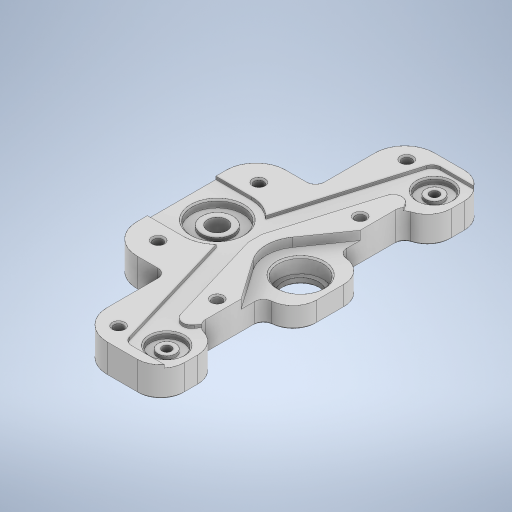
# Autodesk Inventor part: top
Saved by Autodesk Inventor 2023.1 (Build 271208000, 208)
## iProperties
Created: 2023-11-16
Part Number: top
Material: Všeobecné
Document SubType Name: Modeling
Designer: zavrel
Density: 1 g/cm^3
Appearance: Výchozí
Author: zavrel
Autodesk Inventor part; units mm, degrees
ref_plane "YZ Plane" through (0, 0, 0) normal (1, 0, 0) x (0, 1, 0)
ref_plane "XZ Plane" through (0, 0, 0) normal (0, 1, 0) x (-1, 0, 0)
ref_plane "XY Plane" through (0, 0, 0) normal (0, 0, 1) x (1, 0, 0)
sketch "Náčrt1" plane through (0, 0, 0) normal (0, 1, 0) x (-1, 0, 0)
  line L0 (-26.1298, 2.5) -> (-26.1298, 15)
  line L1 (-26.1298, 15) -> (-16.1298, 15)
  line L2 (-16.1298, 15) -> (-16.1298, 37.5)
  line L3 (-16.1298, 37.5) -> (-24.1298, 37.5)
  line L4 (-24.1298, 37.5) -> (-24.1298, 57.5)
  line L5 (-24.1298, 57.5) -> (-16.1298, 57.5)
  line L6 (-16.1298, 57.5) -> (3.8702, 57.5)
  line L7 (3.8702, 57.5) -> (3.8702, 27.5)
  line L8 (3.8702, 27.5) -> (23.8702, 27.5)
  line L9 (23.8702, 27.5) -> (23.8702, 2.5)
  line L10 (23.8702, 2.5) -> (-26.1298, 2.5) construction
  line L11 (-26.1298, 2.5) -> (-26.1298, -10)
  line L12 (-26.1298, -10) -> (-16.1298, -10)
  line L13 (-16.1298, -10) -> (-16.1298, -32.5)
  line L14 (-16.1298, -32.5) -> (-24.1298, -32.5)
  line L15 (-24.1298, -32.5) -> (-24.1298, -52.5)
  line L16 (-24.1298, -52.5) -> (-16.1298, -52.5)
  line L17 (-16.1298, -52.5) -> (3.8702, -52.5)
  line L18 (3.8702, -52.5) -> (3.8702, -22.5)
  line L19 (3.8702, -22.5) -> (23.8702, -22.5)
  line L20 (23.8702, -22.5) -> (23.8702, 2.5)
  circle A0 centre (-16.1298, 47.5) radius 5.5
  line L21 (-24.1298, 47.5) -> (17.4251, 47.5) construction
  circle A1 centre (-16.1298, -42.5) radius 5.5
  line L22 (-24.1298, -42.5) -> (17.4251, -42.5) construction
  circle A2 centre (11.8702, 2.5) radius 8.5
  circle A3 centre (-16.1298, 2.5) radius 7.5
  line L23 (-16.1298, 47.5) -> (-16.1298, -42.5) construction
  point P0 (0, 0)
  point P1 (-26.1298, 8.75)
  point P2 (-16.1298, 2.5)
  dimension "d0" = 25
  dimension "d1" = 50
  dimension "d3" = 20
  dimension "d4" = 8
  dimension "d5" = 20
  dimension "d6" = 20
  dimension "d7" = 11
  dimension "d8" = 90
  dimension "d9" = 8
  dimension "d10" = 17
  dimension "d13" = 15
  dimension "d15" = 12
  dimension "d17" = 10
  constraints: 48 end point, 12 symmetric about line, 9 perpendicular, 8 point on line, 4 centre point, 4 midpoint, 2 vertical, 1 horizontal, 1 other
  measures "d0" distance between parallel lines of L12 L1
  measures "d1" distance between parallel lines of L19 L8
  measures "d3" distance of L3.end L4.end
  measures "d4" distance between parallel lines of L13 L15
  measures "d5" distance between parallel lines of L13 L18
  measures "d6" distance between parallel lines of L18 L20
  measures "d7" diameter of A0
  measures "d8" distance of L23.end L23.start
  measures "d9" distance from line of L4 L23.start
  measures "d10" diameter of A2
  measures "d13" diameter of A3
  measures "d15" distance from line of L9 A2.centre
  measures "d17" distance of L11.end L12.end
extrude "Vysunutí1" add sketch "Náčrt1" along normal blind 10
sketch "Náčrt2" plane through (0, 0, 0) normal (0, -1, 0) x (1, 0, 0)
  line L0 (16.1298, -10) -> (16.1298, -32.5) projected
  line L1 (26.1298, -10) -> (16.1298, -10) projected
  line L2 (26.1298, 15) -> (26.1298, -10) projected
  line L3 (16.1298, 15) -> (26.1298, 15) projected
  line L4 (16.1298, 37.5) -> (16.1298, 15) projected
  line L5 (24.1298, 37.5) -> (16.1298, 37.5) projected
  line L6 (24.1298, 57.5) -> (24.1298, 37.5) projected
  line L7 (-3.8702, 57.5) -> (24.1298, 57.5) projected
  line L8 (-3.8702, 27.5) -> (-3.8702, 57.5) projected
  line L9 (-23.8702, 27.5) -> (-3.8702, 27.5) projected
  line L10 (-23.8702, -22.5) -> (-23.8702, 27.5) projected
  line L11 (-3.8702, -22.5) -> (-23.8702, -22.5) projected
  line L12 (-3.8702, -52.5) -> (-3.8702, -22.5) projected
  line L13 (24.1298, -52.5) -> (-3.8702, -52.5) projected
  line L14 (24.1298, -32.5) -> (24.1298, -52.5) projected
  line L15 (16.1298, -32.5) -> (24.1298, -32.5) projected
  circle A0 centre (16.1298, 47.5) radius 5.5 projected
  circle A1 centre (16.1298, -42.5) radius 5.5 projected
  circle A2 centre (-11.8702, 2.5) radius 8.5 projected
  circle A3 centre (16.1298, 2.5) radius 7.5 projected
  circle A4 centre (16.1298, -42.5) radius 1.5
  circle A5 centre (16.1298, 47.5) radius 5.5 projected
  circle A6 centre (16.1298, 47.5) radius 1.5
  point P0 (0, 0)
  dimension "d20" = 3
  constraints: 2 centre point, 2 coincident, 1 equal radius
  measures "d20" diameter of A6
extrude "Vysunutí2" add sketch "Náčrt2" against normal blind 8 contours A0 | A1
sketch "Náčrt3" plane through (0, 0, 0) normal (0, -1, 0) x (1, 0, 0)
  circle A0 centre (16.1298, 47.5) radius 1.5 projected
  circle A1 centre (16.1298, -42.5) radius 1.5 projected
  line L0 (16.1298, -10) -> (16.1298, -32.5) projected
  line L1 (26.1298, -10) -> (16.1298, -10) projected
  line L2 (26.1298, 15) -> (26.1298, -10) projected
  line L3 (16.1298, 15) -> (26.1298, 15) projected
  line L4 (16.1298, 37.5) -> (16.1298, 15) projected
  line L5 (24.1298, 37.5) -> (16.1298, 37.5) projected
  line L6 (24.1298, 57.5) -> (24.1298, 37.5) projected
  line L7 (-3.8702, 57.5) -> (24.1298, 57.5) projected
  line L8 (-3.8702, 27.5) -> (-3.8702, 57.5) projected
  line L9 (-23.8702, 27.5) -> (-3.8702, 27.5) projected
  line L10 (-23.8702, -22.5) -> (-23.8702, 27.5) projected
  line L11 (-3.8702, -22.5) -> (-23.8702, -22.5) projected
  line L12 (-3.8702, -52.5) -> (-3.8702, -22.5) projected
  line L13 (24.1298, -52.5) -> (-3.8702, -52.5) projected
  line L14 (24.1298, -32.5) -> (24.1298, -52.5) projected
  line L15 (16.1298, -32.5) -> (24.1298, -32.5) projected
  circle A2 centre (-11.8702, 2.5) radius 8.5 projected
  circle A3 centre (16.1298, 2.5) radius 7.5 projected
  circle A4 centre (16.1298, 2.5) radius 6
  point P0 (0, 0)
  dimension "d24" = 12
  constraints: 1 centre point, 1 coincident
  measures "d24" diameter of A4
extrude "Vysunutí3" add sketch "Náčrt3" against normal blind 2 contours A3
sketch "Náčrt4" plane through (0, 0, 0) normal (0, -1, 0) x (1, 0, 0)
  circle A0 centre (16.1298, 2.5) radius 6 projected
  circle A1 centre (16.1298, 47.5) radius 1.5 projected
  circle A2 centre (16.1298, -42.5) radius 1.5 projected
  line L0 (16.1298, -10) -> (16.1298, -32.5) projected
  line L1 (26.1298, -10) -> (16.1298, -10) projected
  line L2 (26.1298, 15) -> (26.1298, -10) projected
  line L3 (16.1298, 15) -> (26.1298, 15) projected
  line L4 (16.1298, 37.5) -> (16.1298, 15) projected
  line L5 (24.1298, 37.5) -> (16.1298, 37.5) projected
  line L6 (24.1298, 57.5) -> (24.1298, 37.5) projected
  line L7 (-3.8702, 57.5) -> (24.1298, 57.5) projected
  line L8 (-3.8702, 27.5) -> (-3.8702, 57.5) projected
  line L9 (-23.8702, 27.5) -> (-3.8702, 27.5) projected
  line L10 (-23.8702, -22.5) -> (-23.8702, 27.5) projected
  line L11 (-3.8702, -22.5) -> (-23.8702, -22.5) projected
  line L12 (-3.8702, -52.5) -> (-3.8702, -22.5) projected
  line L13 (24.1298, -52.5) -> (-3.8702, -52.5) projected
  line L14 (24.1298, -32.5) -> (24.1298, -52.5) projected
  line L15 (16.1298, -32.5) -> (24.1298, -32.5) projected
  circle A3 centre (-11.8702, 2.5) radius 8.5 projected
  circle A4 centre (-11.8702, 2.5) radius 3.25
  point P0 (0, 0)
  dimension "d27" = 6.5
  constraints: 1 centre point, 1 coincident
  measures "d27" diameter of A4
extrude "Vysunutí4" add sketch "Náčrt4" against normal blind 7.5 contours A3
sketch "Náčrt5" plane through (-11.8702, 7.5, 2.5) normal (0, 1, 0) x (1, 0, 0)
  circle A0 centre (0, 0) radius 8.5 projected
  circle A1 centre (0, 0) radius 3.25 projected
  circle A2 centre (0, 0) radius 3.25 projected
  circle A3 centre (0, 0) radius 5.25
  point P0 (11.8702, 2.5)
  dimension "d68" = 2
  constraints: 1 centre point, 1 coincident
  measures "d68" radial gap between concentric circles of A3 A1
extrude "Vysunutí5" cut sketch "Náčrt5" against normal blind 1 contours A0
sketch "Náčrt6" plane through (16.1298, 8, -42.5) normal (0, 1, 0) x (1, 0, 0)
  circle A0 centre (0, -90) radius 5.5 projected
  circle A1 centre (0, -90) radius 1.5 projected
  circle A2 centre (0, 0) radius 5.5 projected
  circle A3 centre (0, 0) radius 1.5 projected
  circle A4 centre (0, -90) radius 1.5 projected
  circle A5 centre (0, -90) radius 3
  circle A6 centre (0, 0) radius 1.5 projected
  circle A7 centre (0, 0) radius 3
  point P0 (-16.1298, -42.5)
  dimension "d33" = 1.5
  constraints: 2 centre point, 2 coincident, 1 equal radius
  measures "d33" radial gap between concentric circles of A5 A1
extrude "Vysunutí6" cut sketch "Náčrt6" against normal blind 1 contours A0 | A2
sketch "Náčrt7" plane through (0, 10, 0) normal (0, 1, 0) x (1, 0, 0)
  line L0 (16.1298, 10) -> (16.1298, 32.5) projected
  line L1 (16.1298, 32.5) -> (24.1298, 32.5) projected
  line L2 (24.1298, 32.5) -> (24.1298, 52.5) projected
  line L3 (24.1298, 52.5) -> (-3.8702, 52.5) projected
  line L4 (-3.8702, 52.5) -> (-3.8702, 22.5) projected
  line L5 (-3.8702, 22.5) -> (-23.8702, 22.5) projected
  line L6 (-23.8702, 22.5) -> (-23.8702, -27.5) projected
  line L7 (-23.8702, -27.5) -> (-3.8702, -27.5) projected
  line L8 (-3.8702, -27.5) -> (-3.8702, -57.5) projected
  line L9 (-3.8702, -57.5) -> (24.1298, -57.5) projected
  line L10 (24.1298, -57.5) -> (24.1298, -37.5) projected
  line L11 (24.1298, -37.5) -> (16.1298, -37.5) projected
  line L12 (16.1298, -37.5) -> (16.1298, -15) projected
  line L13 (16.1298, -15) -> (26.1298, -15) projected
  line L14 (26.1298, -15) -> (26.1298, 10) projected
  line L15 (26.1298, 10) -> (16.1298, 10) projected
  circle A0 centre (16.1298, -47.5) radius 5.5 projected
  circle A1 centre (16.1298, 42.5) radius 5.5 projected
  circle A2 centre (-11.8702, -2.5) radius 8.5 projected
  circle A3 centre (16.1298, -2.5) radius 7.5 projected
  circle A4 centre (16.1298, -47.5) radius 5.5 construction
  line L16 (10.8583, -49.0689) -> (-3.7234, -0.0753) construction
  circle A5 centre (-11.8702, -2.5) radius 8.5 construction
  line L17 (-3.7234, -4.9247) -> (10.8583, 44.0689) construction
  circle A6 centre (16.1298, 42.5) radius 5.5 projected
  line L18 (12.2835, -43.3406) -> (0.8159, -4.8101)
  line L19 (16.1298, -37.5) -> (16.1298, -15) projected
  line L20 (16.1298, -37.5) -> (12.2835, -43.3406)
  line L21 (24.1298, 32.5) -> (24.1298, 52.5) projected
  line L22 (24.1298, -54.5) -> (9.0632, -54.5)
  circle A7 centre (-11.8702, -2.5) radius 11.5
  line L23 (9.0632, -54.5) -> (-3.9358, -10.8244)
  line L24 (0.8159, -2.5) -> (0.8159, -4.8101)
  circle A8 centre (-11.8702, -2.5) radius 3.25 construction
  line L25 (-11.8702, -2.5) -> (16.1298, -2.5) construction
  line L26 (12.2835, 38.3406) -> (0.8159, -0.1899)
  line L27 (16.1298, 32.5) -> (12.2835, 38.3406)
  line L28 (24.1298, 49.5) -> (9.0632, 49.5)
  line L29 (9.0632, 49.5) -> (-3.9358, 5.8244)
  line L30 (0.8159, -2.5) -> (0.8159, -0.1899)
  line L31 (-11.8702, -14) -> (-23.8702, -14)
  line L32 (-23.8702, 22.5) -> (-23.8702, -27.5) projected
  line L33 (-11.8702, 9) -> (-23.8702, 9)
  point P0 (0, 0)
  point P1 (-3.9358, 5.8244)
  dimension "d39" = 3
  dimension "d43" = 3
  dimension "d44" = 3
  constraints: 30 end point, 5 point on circle, 5 symmetric about line, 4 point on line, 4 tangent, 3 horizontal, 3 parallel, 1 centre point, 1 vertical, 6 other
  measures "d39" distance between parallel lines of L16 L18
  measures "d43" distance between parallel lines of L9 L22
  measures "d44" radial gap between concentric circles of A5 A7
extrude "Extrusion7" cut sketch "Náčrt7" against normal blind 1 contours L27 L26 L30 L24 L18 L20 L11 L10 L22 L23 A7 L29 L28 L2 L1 | A7 | A7 L31 L6 L33
sketch "Sketch8" plane through (0, 10, 0) normal (0, 1, 0) x (1, 0, 0)
  line L0 (16.1298, 32.5) -> (12.2835, 38.3406) projected
  line L1 (12.2835, 38.3406) -> (0.8159, -0.1899) projected
  line L2 (0.8159, -0.1899) -> (0.8159, -4.8101) projected
  line L3 (0.8159, -4.8101) -> (12.2835, -43.3406) projected
  line L4 (12.2835, -43.3406) -> (16.1298, -37.5) projected
  line L5 (16.1298, -37.5) -> (16.1298, -15) projected
  line L6 (16.1298, -15) -> (26.1298, -15) projected
  line L7 (26.1298, -15) -> (26.1298, 10) projected
  line L8 (26.1298, 10) -> (16.1298, 10) projected
  line L9 (16.1298, 10) -> (16.1298, 32.5) projected
  circle A0 centre (16.1298, -2.5) radius 7.5 projected
  circle A1 centre (16.1298, -2.5) radius 11.4868
  line L10 (16.1298, 10) -> (16.1298, 32.5) projected
  line L11 (16.1298, 17.5) -> (6.7265, 4.0973)
  line L12 (16.1298, -22.5) -> (6.7265, -9.0973)
  point P0 (0, 0)
  point P1 (18.102, 10)
  point P2 (18.102, -15)
  point P3 (26.1298, 3.152)
  point P4 (26.1298, -8.152)
  dimension "d49" = 20
  constraints: 4 end point, 2 point on circle, 2 point on line, 2 tangent, 1 centre point, 1 equal length
  measures "d49" distance of A0.centre L11.start
extrude "Extrusion8" cut sketch "Sketch8" against normal blind 3 contours L9 L8 L7 A1 L11 | A1 L7 | A1 L7 L6 L5 L12 | A0 picked at (25.2965, -2.5)
sketch "Sketch9" plane through (0, 10, 0) normal (0, 1, 0) x (1, 0, 0)
  line L0 (9.0632, 49.5) -> (24.1298, 49.5) projected
  line L1 (24.1298, 49.5) -> (24.1298, 52.5) projected
  line L2 (24.1298, 52.5) -> (-3.8702, 52.5) projected
  line L3 (-3.8702, 52.5) -> (-3.8702, 22.5) projected
  line L4 (-3.8702, 22.5) -> (-23.8702, 22.5) projected
  line L5 (-23.8702, 22.5) -> (-23.8702, 9) projected
  line L6 (-23.8702, -27.5) -> (-3.8702, -27.5) projected
  line L7 (-3.8702, -27.5) -> (-3.8702, -57.5) projected
  line L8 (-3.8702, -57.5) -> (24.1298, -57.5) projected
  line L9 (24.1298, -57.5) -> (24.1298, -54.5) projected
  line L10 (24.1298, -54.5) -> (9.0632, -54.5) projected
  line L11 (9.0632, -54.5) -> (-3.9358, -10.8244) projected
  arc A0 (-3.9358, 5.8244) -> (-11.8702, 9) centre (-11.8702, -2.5) ccw projected
  line L12 (-3.9358, 5.8244) -> (9.0632, 49.5) projected
  line L13 (16.1298, -22.5) -> (6.7265, -9.0973) projected
  arc A1 (6.7265, 4.0973) -> (6.7265, -9.0973) centre (16.1298, -2.5) ccw projected
  line L14 (6.7265, 4.0973) -> (16.1298, 17.5) projected
  line L15 (16.1298, 17.5) -> (16.1298, 32.5) projected
  line L16 (16.1298, 32.5) -> (12.2835, 38.3406) projected
  line L17 (12.2835, 38.3406) -> (0.8159, -0.1899) projected
  line L18 (0.8159, -0.1899) -> (0.8159, -4.8101) projected
  line L19 (0.8159, -4.8101) -> (12.2835, -43.3406) projected
  line L20 (12.2835, -43.3406) -> (16.1298, -37.5) projected
  line L21 (16.1298, -37.5) -> (16.1298, -22.5) projected
  circle A2 centre (16.1298, -2.5) radius 7.5 projected
  line L22 (26.1298, 10) -> (26.1298, -15) projected
  line L23 (16.1298, 10) -> (26.1298, 10) projected
  line L24 (16.1298, 17.5) -> (16.1298, 10) projected
  line L25 (6.7265, 4.0973) -> (16.1298, 17.5) projected
  arc A3 (6.7265, 4.0973) -> (6.7265, -9.0973) centre (16.1298, -2.5) ccw projected
  line L26 (16.1298, -22.5) -> (6.7265, -9.0973) projected
  line L27 (16.1298, -15) -> (16.1298, -22.5) projected
  line L28 (26.1298, -15) -> (16.1298, -15) projected
  line L29 (12.2835, -43.3406) -> (16.1298, -37.5) projected
  line L30 (0.8159, -4.8101) -> (12.2835, -43.3406) projected
  line L31 (0.8159, -0.1899) -> (0.8159, -4.8101) projected
  line L32 (12.2835, 38.3406) -> (0.8159, -0.1899) projected
  line L33 (16.1298, 32.5) -> (12.2835, 38.3406) projected
  line L34 (24.1298, 32.5) -> (16.1298, 32.5) projected
  line L35 (24.1298, 49.5) -> (24.1298, 32.5) projected
  line L36 (9.0632, 49.5) -> (24.1298, 49.5) projected
  line L37 (-3.9358, 5.8244) -> (9.0632, 49.5) projected
  arc A4 (-11.8702, -14) -> (-3.9358, -10.8244) centre (-11.8702, -2.5) ccw projected
  line L38 (9.0632, -54.5) -> (-3.9358, -10.8244) projected
  line L39 (24.1298, -54.5) -> (9.0632, -54.5) projected
  line L40 (24.1298, -37.5) -> (24.1298, -54.5) projected
  line L41 (16.1298, -37.5) -> (24.1298, -37.5) projected
  circle A5 centre (-11.8702, -2.5) radius 8.5 projected
  circle A6 centre (16.1298, 42.5) radius 5.5 projected
  circle A7 centre (16.1298, -47.5) radius 5.5 projected
  circle A8 centre (3.3734, -50.9251) radius 1.6
  circle A9 centre (12.1298, -26.5254) radius 1.6
  circle A10 centre (-14.8339, -19.4088) radius 1.6
  line L42 (-11.8702, -2.5) -> (16.1298, -2.5) construction
  circle A11 centre (3.3734, 45.9251) radius 1.6
  circle A12 centre (12.1298, 21.5254) radius 1.6
  circle A13 centre (-14.8339, 14.4088) radius 1.6
  arc A14 (-3.9358, 5.8244) -> (-11.8702, 9) centre (-11.8702, -2.5) ccw projected
  line L43 (-23.8702, 9) -> (-11.8702, 9) projected
  line L44 (-23.8702, -14) -> (-23.8702, 9) projected
  line L45 (-11.8702, -14) -> (-23.8702, -14) projected
  line L46 (-23.8702, 9) -> (-11.8702, 9) projected
  line L47 (-11.8702, -14) -> (-23.8702, -14) projected
  line L48 (-23.8702, -14) -> (-23.8702, -27.5) projected
  arc A15 (-11.8702, -14) -> (-3.9358, -10.8244) centre (-11.8702, -2.5) ccw projected
  point P0 (0, 0)
  dimension "d51" = 6.5749
  dimension "d52" = 7.2436
  dimension "d53" = 9.0363
  dimension "d54" = 8.0912
  dimension "d55" = 11.5254
  dimension "d56" = 4
  dimension "d57" = 3.2
  constraints: 6 centre point, 3 symmetric about line, 2 end point, 2 equal radius, 1 horizontal, 3 other
  measures "d51" distance from line of L8 A8.centre
  measures "d52" distance from line of L7 A8.centre
  measures "d53" distance from line of L5 A10.centre
  measures "d54" distance from line of L6 A10.centre
  measures "d55" distance from line of L28 A9.centre
  measures "d56" distance from line of A9.centre L21
  measures "d57" diameter of A10
extrude "Extrusion9" cut sketch "Sketch9" against normal up to surface (10 mm away) contours A8 | A9 | A10 | A11 | A12 | A13
fillet "Fillet1" radius 10 4 edges at (-23.8702, 5, 27.5) (-23.8702, 5, -22.5) (-3.8702, 5, 57.5) (-3.8702, 5, -52.5)
fillet "Fillet2" radius 3 6 edges at (16.1298, 3.5, -10) (16.1298, 4.5, -32.5) (16.1298, 3.5, 15) (16.1298, 4.5, 37.5) (-3.8702, 5, -22.5) (-3.8702, 5, 27.5)
fillet "Fillet3" radius 8 4 edges at (24.1298, 5, 57.5) (24.1298, 4.5, 37.5) (24.1298, 4.5, -32.5) (24.1298, 5, -52.5)
fillet "Fillet4" radius 8 2 edges at (26.1298, 3.5, 15) (26.1298, 3.5, -10)
fillet "Fillet5" radius 3 4 edges at (9.0632, 9.5, 54.5) (12.2835, 9.5, 43.3406) (12.2835, 9.5, -38.3406) (9.0632, 9.5, -49.5)
chamfer "Chamfer1" distance 0.5 angle 45 10 edges at (21.6298, 9, 47.5) (23.6298, 7, 2.5) (-3.3702, 9, 2.5) (21.6298, 9, -42.5) (1.7734, 10, 50.9251) (-16.4339, 10, 19.4088) (-16.4339, 10, -14.4088) (1.7734, 10, -45.9251) (10.5298, 10, -21.5254) (10.5298, 10, 26.5254)
sketch "Sketch10" plane through (0, 0, 0) normal (0, -1, 0) x (1, 0, 0)
  point P0 (0, 0)
sketch "Sketch11" plane through (-23.8702, 9, 14) normal (-1, 0, 0) x (0, 0, 1)
  line L0 (-26.5, -9) -> (-26.5, 1) projected
  line L1 (-26.5, -9) -> (3.5, -9) projected
  line L2 (3.5, 1) -> (3.5, -9) projected
  line L3 (0, 1) -> (3.5, 1) projected
  line L4 (0, 1) -> (0, 0) projected
  line L5 (0, 0) -> (-23, 0) projected
  line L6 (-23, 0) -> (-23, 1) projected
  line L7 (-26.5, 1) -> (-23, 1) projected
  line L8 (3.5, 1) -> (3.5, -9) construction
  line L9 (3.5, -4) -> (-26.5, -4) construction
  line L10 (-26.5, -9) -> (-26.5, 1) construction
  line L11 (-6.9545, -9) -> (-16.0455, -9) construction
  line L12 (-11.5, -9) -> (-11.5, 1) construction
  line L13 (-18.0973, 1) -> (-4.9027, 1) construction
  circle A0 centre (-0.5, -4) radius 1.6
  circle A1 centre (-22.5, -4) radius 1.6
  line L14 (-0.5, -4) -> (-0.5, -1.1985) construction
  line L15 (-0.5, -1.7373) -> (0.6314, -2.8686)
  line L16 (-0.5, -1.7373) -> (-1.6314, -2.8686)
  line L17 (-22.5, -1.7373) -> (-23.6314, -2.8686)
  line L18 (-22.5, -1.7373) -> (-21.3686, -2.8686)
  point P0 (-14, -9)
  point P1 (-21.3686, -2.8686)
  dimension "d69" = 3.2
  dimension "d70" = 22
  dimension "d91" = 90
  constraints: 14 end point, 4 midpoint, 4 symmetric about line, 2 centre point, 2 point on circle, 2 point on line, 2 tangent, 1 vertical, 1 other
  measures "d69" diameter of A0
  measures "d70" distance of A1.centre L14.start
  measures "d91" angle of L16 L15
sketch "Sketch12" plane through (0, 0, 0) normal (0, -1, 0) x (1, 0, 0)
  arc A0 (18.8571, -10.0124) -> (26.1298, -2.0455) centre (18.1298, -2.0455) ccw projected
  line L0 (26.1298, 7.0455) -> (26.1298, -2.0455) projected
  arc A1 (26.1298, 7.0455) -> (18.8571, 15.0124) centre (18.1298, 7.0455) ccw projected
  arc A2 (16.1298, 18) -> (18.8571, 15.0124) centre (19.1298, 18) ccw projected
  line L1 (16.1298, 34.5) -> (16.1298, 18) projected
  arc A3 (18.3116, 37.3863) -> (16.1298, 34.5) centre (19.1298, 34.5) ccw projected
  arc A4 (18.3116, 37.3863) -> (24.1298, 45.083) centre (16.1298, 45.083) ccw projected
  line L2 (24.1298, 49.5) -> (24.1298, 45.083) projected
  arc A5 (24.1298, 49.5) -> (16.1298, 57.5) centre (16.1298, 49.5) ccw projected
  line L3 (6.1298, 57.5) -> (16.1298, 57.5) projected
  arc A6 (6.1298, 57.5) -> (-3.8702, 47.5) centre (6.1298, 47.5) ccw projected
  line L4 (-3.8702, 30.5) -> (-3.8702, 47.5) projected
  arc A7 (-6.8702, 27.5) -> (-3.8702, 30.5) centre (-6.8702, 30.5) ccw projected
  line L5 (-13.8702, 27.5) -> (-6.8702, 27.5) projected
  arc A8 (-13.8702, 27.5) -> (-23.8702, 17.5) centre (-13.8702, 17.5) ccw projected
  line L6 (-23.8702, -12.5) -> (-23.8702, 17.5) projected
  arc A9 (-23.8702, -12.5) -> (-13.8702, -22.5) centre (-13.8702, -12.5) ccw projected
  line L7 (-6.8702, -22.5) -> (-13.8702, -22.5) projected
  arc A10 (-3.8702, -25.5) -> (-6.8702, -22.5) centre (-6.8702, -25.5) ccw projected
  line L8 (-3.8702, -42.5) -> (-3.8702, -25.5) projected
  arc A11 (-3.8702, -42.5) -> (6.1298, -52.5) centre (6.1298, -42.5) ccw projected
  line L9 (16.1298, -52.5) -> (6.1298, -52.5) projected
  arc A12 (16.1298, -52.5) -> (24.1298, -44.5) centre (16.1298, -44.5) ccw projected
  line L10 (24.1298, -40.083) -> (24.1298, -44.5) projected
  arc A13 (24.1298, -40.083) -> (18.3116, -32.3863) centre (16.1298, -40.083) ccw projected
  arc A14 (16.1298, -29.5) -> (18.3116, -32.3863) centre (19.1298, -29.5) ccw projected
  line L11 (16.1298, -13) -> (16.1298, -29.5) projected
  arc A15 (18.8571, -10.0124) -> (16.1298, -13) centre (19.1298, -13) ccw projected
  circle A16 centre (3.3734, -45.9251) radius 1.6 projected
  circle A17 centre (-14.8339, -14.4088) radius 1.6 projected
  circle A18 centre (3.3734, 50.9251) radius 1.6 projected
  circle A19 centre (-14.8339, 19.4088) radius 1.6 projected
  circle A20 centre (12.1298, -21.5254) radius 1.6 projected
  circle A21 centre (12.1298, 26.5254) radius 1.6 projected
  circle A22 centre (-11.8702, 2.5) radius 3.25 projected
  circle A23 centre (16.1298, 2.5) radius 6 projected
  circle A24 centre (16.1298, 47.5) radius 1.5 projected
  circle A25 centre (16.1298, -42.5) radius 1.5 projected
  circle A26 centre (-11.8702, 2.5) radius 3.25 projected
  line L12 (-11.8702, 2.5) -> (-23.8702, 2.5) construction
  line L13 (-23.8702, 14) -> (-23.8702, -9) projected
  line L14 (-20.8702, 10.5) -> (-18.8702, 10.5)
  line L15 (-18.8702, 10.5) -> (-18.8702, 16.5)
  line L16 (-18.8702, 16.5) -> (-20.8702, 16.5)
  line L17 (-20.8702, 16.5) -> (-20.8702, 10.5)
  line L18 (-20.8702, 10.5) -> (-18.8702, 16.5) construction
  line L19 (-18.8702, 10.5) -> (-20.8702, 16.5) construction
  line L20 (-20.8702, -5.5) -> (-18.8702, -5.5)
  line L21 (-18.8702, -5.5) -> (-18.8702, -11.5)
  line L22 (-18.8702, -11.5) -> (-20.8702, -11.5)
  line L23 (-20.8702, -11.5) -> (-20.8702, -5.5)
  line L24 (-20.8702, -5.5) -> (-18.8702, -11.5) construction
  line L25 (-18.8702, -5.5) -> (-20.8702, -11.5) construction
  point P0 (0, 0)
  point P1 (-19.8702, 13.5)
  point P2 (-19.8702, 16.5)
  point P3 (-19.8702, 10.5)
  point P4 (-19.8702, -8.5)
  point P5 (-19.8702, -11.5)
  point P6 (-19.8702, -5.5)
  point P7 (-19.8702, -8.5)
  dimension "d71" = 6
  dimension "d72" = 3
  dimension "d73" = 22
  dimension "d74" = 2
  constraints: 26 end point, 7 symmetric about line, 6 midpoint, 2 parallel, 1 horizontal, 1 perpendicular
  measures "d71" distance of point (-19.87, 16.5) point (-19.87, 10.5)
  measures "d72" distance between parallel lines of L13 L17
  measures "d73" distance of point (-19.87, -8.5) point (-19.87, 13.5)
  measures "d74" distance between parallel lines of L17 L15
extrude "Extrusion10" cut sketch "Sketch11" against normal blind 16 contours A0 | A0 L16 L15 | A1 | A1 L17 L18
extrude "Extrusion11" cut sketch "Sketch12" against normal blind 8 contours L17 L16 L15 L14 | L20 L21 L22 L23
sketch "Sketch13" plane through (0, 0, 0) normal (0, -1, 0) x (1, 0, 0)
  line L0 (-18.8702, -5.5) -> (-18.8702, -11.5) projected
  line L1 (-18.8702, -11.5) -> (-20.8702, -11.5) projected
  line L2 (-20.8702, -11.5) -> (-20.8702, -5.5) projected
  line L3 (-20.8702, -5.5) -> (-18.8702, -5.5) projected
  line L4 (-20.8702, 16.5) -> (-18.8702, 16.5) projected
  line L5 (-18.8702, 16.5) -> (-18.8702, 10.5) projected
  line L6 (-18.8702, 10.5) -> (-20.8702, 10.5) projected
  line L7 (-20.8702, 10.5) -> (-20.8702, 16.5) projected
  arc A0 (18.8571, -10.0124) -> (26.1298, -2.0455) centre (18.1298, -2.0455) ccw projected
  line L8 (26.1298, 7.0455) -> (26.1298, -2.0455) projected
  arc A1 (26.1298, 7.0455) -> (18.8571, 15.0124) centre (18.1298, 7.0455) ccw projected
  arc A2 (16.1298, 18) -> (18.8571, 15.0124) centre (19.1298, 18) ccw projected
  line L9 (16.1298, 34.5) -> (16.1298, 18) projected
  arc A3 (18.3116, 37.3863) -> (16.1298, 34.5) centre (19.1298, 34.5) ccw projected
  arc A4 (18.3116, 37.3863) -> (24.1298, 45.083) centre (16.1298, 45.083) ccw projected
  line L10 (24.1298, 49.5) -> (24.1298, 45.083) projected
  arc A5 (24.1298, 49.5) -> (16.1298, 57.5) centre (16.1298, 49.5) ccw projected
  line L11 (6.1298, 57.5) -> (16.1298, 57.5) projected
  arc A6 (6.1298, 57.5) -> (-3.8702, 47.5) centre (6.1298, 47.5) ccw projected
  line L12 (-3.8702, 30.5) -> (-3.8702, 47.5) projected
  arc A7 (-6.8702, 27.5) -> (-3.8702, 30.5) centre (-6.8702, 30.5) ccw projected
  line L13 (-13.8702, 27.5) -> (-6.8702, 27.5) projected
  arc A8 (-13.8702, 27.5) -> (-23.8702, 17.5) centre (-13.8702, 17.5) ccw projected
  line L14 (-23.8702, -12.5) -> (-23.8702, 17.5) projected
  arc A9 (-23.8702, -12.5) -> (-13.8702, -22.5) centre (-13.8702, -12.5) ccw projected
  line L15 (-6.8702, -22.5) -> (-13.8702, -22.5) projected
  arc A10 (-3.8702, -25.5) -> (-6.8702, -22.5) centre (-6.8702, -25.5) ccw projected
  line L16 (-3.8702, -42.5) -> (-3.8702, -25.5) projected
  arc A11 (-3.8702, -42.5) -> (6.1298, -52.5) centre (6.1298, -42.5) ccw projected
  line L17 (16.1298, -52.5) -> (6.1298, -52.5) projected
  arc A12 (16.1298, -52.5) -> (24.1298, -44.5) centre (16.1298, -44.5) ccw projected
  line L18 (24.1298, -40.083) -> (24.1298, -44.5) projected
  arc A13 (24.1298, -40.083) -> (18.3116, -32.3863) centre (16.1298, -40.083) ccw projected
  arc A14 (16.1298, -29.5) -> (18.3116, -32.3863) centre (19.1298, -29.5) ccw projected
  line L19 (16.1298, -13) -> (16.1298, -29.5) projected
  arc A15 (18.8571, -10.0124) -> (16.1298, -13) centre (19.1298, -13) ccw projected
  circle A16 centre (3.3734, -45.9251) radius 1.6 projected
  circle A17 centre (-14.8339, -14.4088) radius 1.6 projected
  circle A18 centre (3.3734, 50.9251) radius 1.6 projected
  circle A19 centre (-14.8339, 19.4088) radius 1.6 projected
  circle A20 centre (12.1298, -21.5254) radius 1.6 projected
  circle A21 centre (12.1298, 26.5254) radius 1.6 projected
  circle A22 centre (-11.8702, 2.5) radius 3.25 projected
  circle A23 centre (16.1298, 2.5) radius 6 projected
  circle A24 centre (16.1298, 47.5) radius 1.5 projected
  circle A25 centre (16.1298, -42.5) radius 1.5 projected
  circle A26 centre (12.1298, 26.5254) radius 1.6 projected
  circle A27 centre (12.1298, 26.5254) radius 3
  circle A28 centre (16.1298, 47.5) radius 3
  circle A29 centre (3.3734, 50.9251) radius 3
  circle A30 centre (-14.8339, 19.4088) radius 3
  point P0 (0, 0)
  dimension "d79" = 6
  constraints: 4 centre point, 3 equal radius, 1 coincident
  measures "d79" diameter of A27
extrude "Extrusion12" cut sketch "Sketch13" against normal blind 3 contours A27 | A28 | A29 | A30
sketch "Sketch14" plane through (0, 0, 0) normal (0, -1, 0) x (1, 0, 0)
  circle A0 centre (3.3734, 50.9251) radius 3 projected
  circle A1 centre (12.1298, 26.5254) radius 3 projected
  circle A2 centre (-14.8339, 19.4088) radius 3 projected
  circle A3 centre (16.1298, 47.5) radius 3 projected
  line L0 (-18.8702, -5.5) -> (-18.8702, -11.5) projected
  line L1 (-18.8702, -11.5) -> (-20.8702, -11.5) projected
  line L2 (-20.8702, -11.5) -> (-20.8702, -5.5) projected
  line L3 (-20.8702, -5.5) -> (-18.8702, -5.5) projected
  line L4 (-20.8702, 16.5) -> (-18.8702, 16.5) projected
  line L5 (-18.8702, 16.5) -> (-18.8702, 10.5) projected
  line L6 (-18.8702, 10.5) -> (-20.8702, 10.5) projected
  line L7 (-20.8702, 10.5) -> (-20.8702, 16.5) projected
  arc A4 (18.8571, -10.0124) -> (26.1298, -2.0455) centre (18.1298, -2.0455) ccw projected
  line L8 (26.1298, 7.0455) -> (26.1298, -2.0455) projected
  arc A5 (26.1298, 7.0455) -> (18.8571, 15.0124) centre (18.1298, 7.0455) ccw projected
  arc A6 (16.1298, 18) -> (18.8571, 15.0124) centre (19.1298, 18) ccw projected
  line L9 (16.1298, 34.5) -> (16.1298, 18) projected
  arc A7 (18.3116, 37.3863) -> (16.1298, 34.5) centre (19.1298, 34.5) ccw projected
  arc A8 (18.3116, 37.3863) -> (24.1298, 45.083) centre (16.1298, 45.083) ccw projected
  line L10 (24.1298, 49.5) -> (24.1298, 45.083) projected
  arc A9 (24.1298, 49.5) -> (16.1298, 57.5) centre (16.1298, 49.5) ccw projected
  line L11 (6.1298, 57.5) -> (16.1298, 57.5) projected
  arc A10 (6.1298, 57.5) -> (-3.8702, 47.5) centre (6.1298, 47.5) ccw projected
  line L12 (-3.8702, 30.5) -> (-3.8702, 47.5) projected
  arc A11 (-6.8702, 27.5) -> (-3.8702, 30.5) centre (-6.8702, 30.5) ccw projected
  line L13 (-13.8702, 27.5) -> (-6.8702, 27.5) projected
  arc A12 (-13.8702, 27.5) -> (-23.8702, 17.5) centre (-13.8702, 17.5) ccw projected
  line L14 (-23.8702, -12.5) -> (-23.8702, 17.5) projected
  arc A13 (-23.8702, -12.5) -> (-13.8702, -22.5) centre (-13.8702, -12.5) ccw projected
  line L15 (-6.8702, -22.5) -> (-13.8702, -22.5) projected
  arc A14 (-3.8702, -25.5) -> (-6.8702, -22.5) centre (-6.8702, -25.5) ccw projected
  line L16 (-3.8702, -42.5) -> (-3.8702, -25.5) projected
  arc A15 (-3.8702, -42.5) -> (6.1298, -52.5) centre (6.1298, -42.5) ccw projected
  line L17 (16.1298, -52.5) -> (6.1298, -52.5) projected
  arc A16 (16.1298, -52.5) -> (24.1298, -44.5) centre (16.1298, -44.5) ccw projected
  line L18 (24.1298, -40.083) -> (24.1298, -44.5) projected
  arc A17 (24.1298, -40.083) -> (18.3116, -32.3863) centre (16.1298, -40.083) ccw projected
  arc A18 (16.1298, -29.5) -> (18.3116, -32.3863) centre (19.1298, -29.5) ccw projected
  line L19 (16.1298, -13) -> (16.1298, -29.5) projected
  arc A19 (18.8571, -10.0124) -> (16.1298, -13) centre (19.1298, -13) ccw projected
  circle A20 centre (3.3734, -45.9251) radius 1.6 projected
  circle A21 centre (-14.8339, -14.4088) radius 1.6 projected
  circle A22 centre (12.1298, -21.5254) radius 1.6 projected
  circle A23 centre (-11.8702, 2.5) radius 3.25 projected
  circle A24 centre (16.1298, 2.5) radius 6 projected
  circle A25 centre (16.1298, -42.5) radius 1.5 projected
  line L20 (8.9544, -21.5254) -> (10.5421, -18.7754)
  line L21 (10.5421, -18.7754) -> (13.7175, -18.7754)
  line L22 (13.7175, -18.7754) -> (15.3052, -21.5254)
  line L23 (15.3052, -21.5254) -> (13.7175, -24.2754)
  line L24 (13.7175, -24.2754) -> (10.5421, -24.2754)
  line L25 (10.5421, -24.2754) -> (8.9544, -21.5254)
  line L26 (12.9544, -42.5) -> (14.5421, -39.75)
  line L27 (14.5421, -39.75) -> (17.7175, -39.75)
  line L28 (17.7175, -39.75) -> (19.3052, -42.5)
  line L29 (19.3052, -42.5) -> (17.7175, -45.25)
  line L30 (17.7175, -45.25) -> (14.5421, -45.25)
  line L31 (14.5421, -45.25) -> (12.9544, -42.5)
  line L32 (0.198, -45.9251) -> (1.7857, -43.1751)
  line L33 (1.7857, -43.1751) -> (4.9612, -43.1751)
  line L34 (4.9612, -43.1751) -> (6.5489, -45.9251)
  line L35 (6.5489, -45.9251) -> (4.9612, -48.6751)
  line L36 (4.9612, -48.6751) -> (1.7857, -48.6751)
  line L37 (1.7857, -48.6751) -> (0.198, -45.9251)
  line L38 (-18.0093, -14.4088) -> (-16.4216, -11.6588)
  line L39 (-16.4216, -11.6588) -> (-13.2462, -11.6588)
  line L40 (-13.2462, -11.6588) -> (-11.6585, -14.4088)
  line L41 (-11.6585, -14.4088) -> (-13.2462, -17.1588)
  line L42 (-13.2462, -17.1588) -> (-16.4216, -17.1588)
  line L43 (-16.4216, -17.1588) -> (-18.0093, -14.4088)
  point P0 (0, 0)
  point P1 (-14.8339, -14.4088)
  dimension "d82" = 5.5
  constraints: 48 end point, 3 equal length, 1 coincident, 52 other
  measures "d82" distance between parallel lines of L24 L21
extrude "Extrusion13" cut sketch "Sketch14" against normal blind 2.5 contours L20 L21 L22 L23 L24 L25 | L26 L27 L28 L29 L30 L31 | L32 L33 L34 L35 L36 L37 | L38 L39 L40 L41 L42 L43
chamfer "Chamfer2" distance 0.5 angle 45 42 edges at (13.1298, 0, 47.5) (22.5116, 0, 40.2588) (16.7366, 0, 36.3091) (16.1298, 0, 26.25) (16.9142, 0, 15.9774) (24.0382, 0, 12.4391) (26.1298, 0, 2.5) (24.0382, 0, -7.4391) (16.9142, 0, -10.9774) (16.1298, 0, -21.25) (16.7366, 0, -31.3091) (22.5116, 0, -35.2588) (24.1298, 0, -42.2915) (21.7867, 0, -50.1569) (11.1298, 0, -52.5) (-0.9413, 0, -49.5711) (-3.8702, 0, -34) (-4.7489, 0, -23.3787) (-10.3702, 0, -22.5) (-20.9413, 0, -19.5711) (-23.8702, 0, 2.5) (-20.9413, 0, 24.5711) (-10.3702, 0, 27.5) (-4.7489, 0, 28.3787) (-3.8702, 0, 39) (-0.9413, 0, 54.5711) (11.1298, 0, 57.5) (21.7867, 0, 55.1569) (24.1298, 0, 47.2915) (10.1298, 0, 2.5) (9.1298, 0, 26.5254) (-17.8339, 0, 19.4088) (-15.1202, 0, 2.5) (-18.8702, 0, 13.5) (-19.8702, 0, 10.5) (-19.8702, 0, 16.5) (-20.8702, 0, 13.5) (-18.8702, 0, -8.5) (-19.8702, 0, -11.5) (-20.8702, 0, -8.5) (-19.8702, 0, -5.5) (0.3734, 0, 50.9251)
